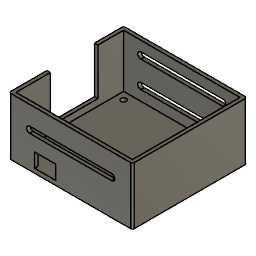
tempbox (Autodesk Fusion 360 design; units mm, degrees)
Autodesk Fusion 360 part; units mm, degrees
sketch "Sketch1" plane through (0, 0, 0) normal (0, 0, 1) x (1, 0, 0)
  line L0 (0, 0) -> (70, 0)
  line L1 (70, 0) -> (70, 65)
  line L2 (70, 65) -> (0, 65)
  line L3 (0, 65) -> (0, 0)
  dimension "d1" = 70
  dimension "d2" = 65
  constraint horizontal L0
  constraint vertical L1
  constraint horizontal L2
  constraint vertical L3
  constraint coincident L0.start L3.end
  measures "d1" distance of L0.start L0.end
  measures "d2" distance of L0.start L2.end
extrude "Extrude1" add sketch "Sketch1" along normal blind 2.5
sketch "Sketch2" plane through (0, 0, 2.5) normal (0, 0, 1) x (-1, 0, 0)
  line L0 (0, -65) -> (0, 0)
  line L1 (0, 0) -> (-70, 0)
  line L2 (-70, 0) -> (-70, -65)
  line L3 (-70, -65) -> (0, -65)
  line L4 (0, -65) -> (-2, -65)
  line L5 (-2, -65) -> (-2, 0)
  line L6 (-2, 0) -> (0, 0)
  line L7 (0, 0) -> (0, -65)
  line L8 (-70, -65) -> (-68, -65)
  line L9 (-68, -65) -> (-68, 0)
  line L10 (-68, 0) -> (-70, 0)
  line L11 (-70, 0) -> (-70, -65)
  line L12 (0, -65) -> (-70, -65)
  line L13 (-70, -65) -> (-70, -63)
  line L14 (-70, -63) -> (0, -63)
  line L15 (0, -63) -> (0, -65)
  line L16 (0, 0) -> (-70, 0)
  line L17 (-70, 0) -> (-70, -2)
  line L18 (-70, -2) -> (0, -2)
  line L19 (0, -2) -> (0, 0)
  dimension "d5" = 2
  dimension "d6" = 2
  dimension "d7" = 65
  dimension "d8" = 2
  dimension "d9" = 2
  constraint horizontal L4
  constraint vertical L5
  constraint horizontal L6
  constraint vertical L7
  constraint coincident L0.start L3.end
  constraint horizontal L8
  constraint vertical L9
  constraint horizontal L10
  constraint vertical L11
  constraint coincident L2.end L3.start
  constraint horizontal L12
  constraint vertical L13
  constraint horizontal L14
  constraint vertical L15
  constraint horizontal L16
  constraint vertical L17
  constraint horizontal L18
  constraint vertical L19
  constraint coincident L0.end L1.start
  measures "d5" distance of L0.start L4.end
  measures "d6" distance of L2.end L8.end
  measures "d7" distance of L2.end L1.end
  measures "d8" distance of L0.start L14.end
  measures "d9" distance of L0.end L18.end
extrude "Extrude2" add sketch "Sketch2" along normal blind 30 contours L0 L3 L4 L5 L7 L12 L14 L15 | L0 L5 L7 L14 L18 | L3 L5 L9 L12 L14 | L0 L1 L5 L6 L7 L16 L18 L19 | L2 L3 L8 L9 L11 L12 L13 L14 | L1 L5 L9 L16 L18 | L2 L9 L11 L14 L18 | L1 L2 L9 L10 L11 L16 L17 L18
sketch "Sketch3" plane through (0, 0, 2.5) normal (0, 0, 1) x (-1, 0, 0)
  line L0 (-2, -2) -> (-68, -2)
  line L1 (-68, -2) -> (-68, -63)
  line L2 (-68, -63) -> (-2, -63)
  line L3 (-2, -63) -> (-2, -2)
  circle A0 centre (-6.2, -6.3) radius 1.5
  circle A1 centre (-6.2, -58.8) radius 1.5
  circle A2 centre (-64.77, -58.8) radius 1.5
  circle A3 centre (-64.77, -6.3) radius 1.5
  dimension "d12" = 3
  dimension "d13" = 3
  dimension "d14" = 3
  dimension "d15" = 3
  dimension "d16" = 58.57
  dimension "d17" = 58.57
  dimension "d18" = 52.5
  dimension "d19" = 52.5
  measures "d12" diameter of A0
  measures "d13" diameter of A1
  measures "d14" diameter of A2
  measures "d15" diameter of A3
  measures "d16" distance of A0.centre A3.centre
  measures "d17" distance of A1.centre A2.centre
  measures "d18" distance of A0.centre A1.centre
  measures "d19" distance of A2.centre A3.centre
extrude "Extrude3" cut sketch "Sketch3" against normal blind 2.5 contours A0 | A1 | A2 | A3
sketch "Sketch6" plane through (0, 0, 0) normal (0, -1, 0) x (1, 0, 0)
  line L0 (0, 0) -> (70, 0)
  line L1 (70, 0) -> (70, 32.5)
  line L2 (70, 32.5) -> (0, 32.5)
  line L3 (0, 32.5) -> (0, 0)
  line L4 (14.5, 2.5) -> (26.5, 2.5)
  line L5 (26.5, 2.5) -> (26.5, 10.5)
  line L6 (26.5, 10.5) -> (14.5, 10.5)
  line L7 (14.5, 10.5) -> (14.5, 2.5)
  line L8 (11.75, 18.25) -> (58.25, 18.25)
  arc A0 (58.25, 18.25) -> (58.25, 21.75) centre (58.25, 20) ccw
  line L9 (58.25, 21.75) -> (11.75, 21.75)
  arc A1 (11.75, 21.75) -> (11.75, 18.25) centre (11.75, 20) ccw
  line L10 (10, 20) -> (60, 20) construction
  dimension "d32" = 12
  dimension "d33" = 8
  dimension "d34" = 2.5
  dimension "d35" = 14.5
  dimension "d36" = 3.5
  constraint horizontal L4
  constraint vertical L5
  constraint horizontal L6
  constraint vertical L7
  constraint tangent L8 A0
  constraint tangent A0 L9
  constraint parallel L8 L9
  constraint tangent L9 A1
  constraint tangent L8 A1
  constraint midpoint A1 L10.start
  constraint midpoint A0 L10.end
  constraint horizontal L10
  measures "d32" distance of L4.start L4.end
  measures "d33" distance of L4.start L6.end
  measures "d34" distance of L0 L4
  measures "d35" distance of L3 L7
  measures "d36" diameter of A0
sketch "Sketch7" plane through (0, 0, 0) normal (-1, 0, 0) x (0, -1, 0)
  line L0 (-65, 0) -> (0, 0)
  line L1 (0, 0) -> (0, 32.5)
  line L2 (0, 32.5) -> (-65, 32.5)
  line L3 (-65, 32.5) -> (-65, 0)
  line L4 (-48.5, 6.2) -> (-21.5, 6.2)
  line L5 (-21.5, 6.2) -> (-21.5, 32.5)
  line L6 (-21.5, 32.5) -> (-48.5, 32.5)
  line L7 (-48.5, 32.5) -> (-48.5, 6.2)
  dimension "d37" = 16.5
  dimension "d38" = 6.2
  dimension "d47" = 27
  dimension "d48" = 26.3
  constraint horizontal L4
  constraint vertical L5
  constraint horizontal L6
  constraint vertical L7
  measures "d37" distance of L3 L7
  measures "d38" distance of L0 L4
  measures "d47" distance of L4.start L4.end
  measures "d48" distance of L4 L6
extrude "Extrude6" cut sketch "Sketch7" against normal blind 2 contours L2 L4 L5 L6 L7
extrude "Extrude7" cut sketch "Sketch6" against normal blind 2 contours L4 L5 L6 L7 | L8 A0 L9 A1
sketch "Sketch8" plane through (0, 65, 0) normal (0, 1, 0) x (-1, 0, 0)
  line L0 (-70, 0) -> (0, 0)
  line L1 (0, 0) -> (0, 32.5)
  line L2 (0, 32.5) -> (-70, 32.5)
  line L3 (-70, 32.5) -> (-70, 0)
  line L4 (-58.25, 23.25) -> (-11.75, 23.25)
  arc A0 (-11.75, 23.25) -> (-11.75, 26.75) centre (-11.75, 25) ccw
  line L5 (-11.75, 26.75) -> (-58.25, 26.75)
  arc A1 (-58.25, 26.75) -> (-58.25, 23.25) centre (-58.25, 25) ccw
  line L6 (-60, 25) -> (-10, 25) construction
  line L7 (-58.25, 8.25) -> (-11.75, 8.25)
  arc A2 (-11.75, 8.25) -> (-11.75, 11.75) centre (-11.75, 10) ccw
  line L8 (-11.75, 11.75) -> (-58.25, 11.75)
  arc A3 (-58.25, 11.75) -> (-58.25, 8.25) centre (-58.25, 10) ccw
  line L9 (-60, 10) -> (-10, 10) construction
  dimension "d43" = 3.5
  dimension "d44" = 3.5
  constraint tangent L4 A0
  constraint tangent A0 L5
  constraint parallel L4 L5
  constraint tangent L5 A1
  constraint tangent L4 A1
  constraint midpoint A1 L6.start
  constraint midpoint A0 L6.end
  constraint horizontal L6
  constraint tangent L7 A2
  constraint tangent A2 L8
  constraint parallel L7 L8
  constraint tangent L8 A3
  constraint tangent L7 A3
  constraint midpoint A3 L9.start
  constraint midpoint A2 L9.end
  constraint horizontal L9
  measures "d43" diameter of A0
  measures "d44" diameter of A2
extrude "Extrude8" cut sketch "Sketch8" against normal blind 2 contours L4 A0 L5 A1 | L7 A2 L8 A3
fillet "Fillet1" radius 1 4 edges at (70, 0, 16.25) (0, 0, 16.25) (70, 65, 16.25) (0, 65, 16.25)
